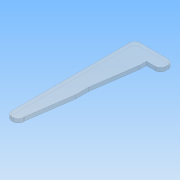
# Autodesk Inventor part: Pin
Saved by Autodesk Inventor 2016 (Build 200138000, 138)
## iProperties
Created: 2016-04-04
Part Number: Pin
Material: Polycarbonate, Clear
Document SubType Name: Modeling
Designer: admin
Density: 1.2 g/cm^3
Appearance: Polycarbonate - Clear
Author: admin
Autodesk Inventor part; units mm, degrees
ref_plane "YZ Plane" through (0, 0, 0) normal (1, 0, 0) x (0, 1, 0)
ref_plane "XZ Plane" through (0, 0, 0) normal (0, 1, 0) x (-1, 0, 0)
ref_plane "XY Plane" through (0, 0, 0) normal (0, 0, 1) x (1, 0, 0)
sketch "Sketch1" plane through (0, 0, 0) normal (0, 0, 1) x (1, 0, 0)
  line L0 (11, 50) -> (-11, 50)
  line L1 (-15, 46) -> (-15, -46)
  line L2 (-11, -50) -> (-10, -50)
  line L3 (-6, -46) -> (-6, -45)
  line L4 (-6, -45) -> (-1, -10)
  line L5 (-1, -10) -> (-1, 0)
  line L6 (-1, 0) -> (4, 35)
  line L7 (4, 35) -> (4, 40)
  arc A0 (-10, -50) -> (-6, -46) centre (-10, -46) ccw
  arc A1 (-15, -46) -> (-11, -50) centre (-11, -46) ccw
  arc A2 (-11, 50) -> (-15, 46) centre (-11, 46) ccw
  line L8 (4, 40) -> (11, 40)
  line L9 (15, 44) -> (15, 46)
  arc A3 (15, 46) -> (11, 50) centre (11, 46) ccw
  arc A4 (11, 40) -> (15, 44) centre (11, 44) ccw
  point P0 (0, 0)
  point P1 (-15, 50)
  point P2 (-15, -50)
  point P3 (-6, -50)
  point P4 (-15, 0)
  point P5 (0, 50)
  dimension "d0" = 19
  dimension "d1" = 14
  dimension "d2" = 100
  dimension "d3" = 9
  dimension "d4" = 4
  dimension "d5" = 4
  dimension "d6" = 30
  dimension "d7" = 45
  dimension "d9" = 10
  dimension "d10" = 5
  constraints: 20 end point, 10 point on circle, 10 tangent, 6 point on line, 5 centre point, 4 perpendicular, 3 equal radius, 2 horizontal, 2 midpoint, 2 parallel, 1 horizontal alignment, 1 vertical alignment
  measures "d0" distance between parallel lines of L7 L1
  measures "d1" distance between parallel lines of L5 L1
  measures "d2" distance of point (-15, 50) point (-15, -50)
  measures "d3" distance of point (-15, -50) point (-6, -50)
  measures "d4" radius of A0
  measures "d5" radius of A3
  measures "d6" distance between parallel lines of L9 L1
  measures "d7" vertical distance of L4.end L6.end
  measures "d9" distance between parallel lines of L0 L8
  measures "d10" distance of L6.end L7.end
extrude "Extrusion1" add sketch "Sketch1" along normal blind 3
body "Solid1"
